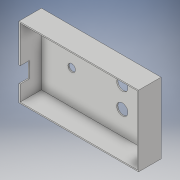
# Autodesk Inventor part: case_top
Saved by Autodesk Inventor 2019 (Build 230136000, 136)
## iProperties
Created: 2019-03-26
Part Number: case_top
Material: Generic
Document SubType Name: Modeling
Designer: janza
Density: 1 g/cm^3
Appearance: Default
Author: janza
Autodesk Inventor part; units mm, degrees
ref_plane "YZ Plane" through (0, 0, 0) normal (1, 0, 0) x (0, 1, 0)
ref_plane "XZ Plane" through (0, 0, 0) normal (0, 1, 0) x (-1, 0, 0)
ref_plane "XY Plane" through (0, 0, 0) normal (0, 0, 1) x (1, 0, 0)
sketch "zakladna" plane through (0, 0, 0) normal (0, 0, 1) x (1, 0, 0)
  line L0 (0, 0) -> (120, 0)
  line L1 (120, 0) -> (120, 70)
  line L2 (120, 70) -> (0, 70)
  line L3 (0, 70) -> (0, 0)
  dimension "d0" = 120
  dimension "d1" = 70
  constraints: 8 end point, 2 parallel, 1 horizontal, 1 perpendicular
  measures "d0" distance of L2.end L1.end
  measures "d1" distance of L1.end L0.end
extrude "Extrusion1" add sketch "zakladna" along normal blind 1.2
sketch "stena_RJ45" plane through (0, 0, 0) normal (0, 0, -1) x (-1, 0, 0)
  line L0 (1.2, 16) -> (0, 16)
  line L1 (0, 16) -> (0, 32.2)
  line L2 (0, 32.2) -> (1.2, 32.2)
  line L3 (1.2, 32.2) -> (1.2, 16)
  line L4 (0, 0) -> (-120, 0) projected
  line L5 (0, 70) -> (0, 0) projected
  dimension "d4" = 1.2
  dimension "d5" = 16.2
  dimension "d6" = 16
  dimension "d7" = 0
  constraints: 8 end point, 2 parallel, 1 horizontal, 1 perpendicular
  measures "d4" distance of L1.end L2.end
  measures "d5" distance of L1.end L0.end
  measures "d6" distance between parallel lines of L4 L0
  measures "d7" distance between parallel lines of L5 L1
sketch "diry_tlacirka_LED" plane through (0, 0, 0) normal (0, 0, -1) x (-1, 0, 0)
  line L0 (-120, 0) -> (-120, 70) projected
  line L1 (-120, 0) -> (-120, 70) projected
  line L2 (-120, 35) -> (-3.6376, 35)
  line L3 (1.2, 32.2) -> (1.2, 16) projected
  line L4 (1.2, 24.1) -> (-82.8, 24.1)
  circle A0 centre (-82.8, 24.1) radius 5.75
  circle A1 centre (-82.8, 45.9) radius 5.75
  circle A2 centre (-31, 35) radius 3.85
  line L5 (0, 70) -> (0, 0) projected
  dimension "d8" = 84
  dimension "d9" = 11.5
  dimension "d10" = 7.7
  dimension "d11" = 31
  constraints: 4 end point, 3 centre point, 2 horizontal, 2 midpoint, 1 coincident, 1 point on line, 1 symmetric about line, 1 other
  measures "d8" distance of L4.start L4.end
  measures "d9" diameter of A0
  measures "d10" diameter of A2
  measures "d11" distance from line of L5 A2.centre
extrude "Extrusion2" cut sketch "diry_tlacirka_LED" against normal blind 2
sketch "steny" plane through (0, 0, 0) normal (0, 0, -1) x (-1, 0, 0)
  line L0 (1.2, 16) -> (0, 16) projected
  line L1 (0, 32.2) -> (1.2, 32.2) projected
  line L2 (1.2, 32.2) -> (1.2, 70)
  line L3 (1.2, 70) -> (1.2, 71.2)
  line L4 (1.2, 71.2) -> (-120, 71.2)
  line L5 (-120, 70) -> (0, 70) projected
  line L6 (-120, 71.2) -> (-121.2, 71.2)
  line L7 (-121.2, 71.2) -> (-121.2, 0)
  line L8 (-121.2, 0) -> (-121.2, -1.2)
  line L9 (-121.2, -1.2) -> (0, -1.2)
  line L10 (0, 0) -> (-120, 0) projected
  line L11 (0, -1.2) -> (1.2, -1.2)
  line L12 (1.2, -1.2) -> (1.2, 16)
  line L13 (0, 70) -> (0, 0) projected
  line L14 (0, 16) -> (0, 0)
  line L15 (-120, 0) -> (-120, 70) projected
  line L16 (0, 0) -> (-120, 0)
  line L17 (-120, 0) -> (-120, 70)
  line L18 (-120, 70) -> (0, 70)
  line L19 (0, 70) -> (0, 32.2)
  dimension "d14" = 1.2
  dimension "d15" = 1.2
  dimension "d16" = 1.2
  dimension "d17" = 1.2
  constraints: 28 end point, 5 point on line, 4 parallel, 3 perpendicular, 2 collinear, 1 vertical
  measures "d14" distance of L2.end L3.end
  measures "d15" distance of L4.end L6.end
  measures "d16" distance of L7.end L8.end
  measures "d17" distance of L9.end L11.end
extrude "Extrusion3" add sketch "steny" against normal blind 23 contours L12 L11 L9 L8 L7 L6 L4 L3 L2 L1 L13 L5 L15 L10 L0
extrude "Extrusion4" add sketch "stena_RJ45" against normal blind 13.7
body "Solid1"
